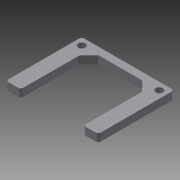
# Autodesk Inventor part: ExtraBoardSpacer
Saved by Autodesk Inventor 2015 (Build 190159000, 159)
## iProperties
Created: 2014-12-16
Part Number: ExtraBoardSpacer
Material: Generic
Document SubType Name: Modeling
Designer: rawrdong
Density: 1 g/cm^3
Appearance: Default
Author: rawrdong
Autodesk Inventor part; units mm, degrees
ref_plane "YZ Plane" through (0, 0, 0) normal (1, 0, 0) x (0, 1, 0)
ref_plane "XZ Plane" through (0, 0, 0) normal (0, 1, 0) x (-1, 0, 0)
ref_plane "XY Plane" through (0, 0, 0) normal (0, 0, 1) x (1, 0, 0)
sketch "Sketch1" plane through (0, 0, 0) normal (0, 0, 1) x (1, 0, 0)
  circle A0 centre (0, 0) radius 1.425
  circle A1 centre (30, 0) radius 1.425
  line L0 (0, 0) -> (30, 0) construction
  line L1 (15, 0) -> (15, -17.6441)
  line L2 (-2.85, 2.85) -> (32.85, 2.85)
  line L3 (32.85, 2.85) -> (32.85, -26.4898)
  line L4 (-2.85, -26.4898) -> (-2.85, 2.85)
  line L5 (2.85, -26.4898) -> (2.85, -3.8397)
  line L6 (2.85, -3.8397) -> (6.5383, 0)
  line L7 (6.5383, 0) -> (23.4617, 0)
  line L8 (23.4617, 0) -> (27.15, -3.8397)
  line L9 (27.15, -3.8397) -> (27.15, -26.4898)
  line L10 (32.85, -26.4898) -> (27.15, -26.4898)
  line L11 (2.85, -26.4898) -> (-2.85, -26.4898)
  dimension "d0" = 2.85
  dimension "d1" = 30
  dimension "d2" = 2.85
  dimension "d3" = 2.85
  dimension "d4" = 2.85
  constraints: 24 end point, 3 parallel, 2 centre point, 2 horizontal, 2 point on line, 2 vertical, 1 coincident, 1 equal radius, 1 horizontal alignment, 1 midpoint, 1 perpendicular, 3 other
  measures "d0" diameter of A1
  measures "d1" distance of L0.end point (0, 0)
  measures "d2" distance from line of L4 L0.start
  measures "d3" distance from line of L2 point (0, 0)
  measures "d4" distance from line of point (0, 0) L5
extrude "Extrusion1" add sketch "Sketch1" along normal blind 3
fillet "Fillet1" radius 1 10 edges at (-2.85, 2.85, 1.5) (32.85, 2.85, 1.5) (-2.85, -26.4898, 1.5) (2.85, -26.4898, 1.5) (32.85, -26.4898, 1.5) (27.15, -26.4898, 1.5) (2.85, -3.8397, 1.5) (6.5383, 0, 1.5) (23.4617, 0, 1.5) (27.15, -3.8397, 1.5)
body "Solid1"
